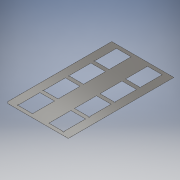
# Autodesk Inventor part: Assembly Stencil
Saved by Autodesk Inventor 2019.4 (Build 234330000, 330)
## iProperties
Created: 2021-01-11
Part Number: Assembly Stencil
Material: Stainless Steel
Document SubType Name: Modeling
Designer: caleb
Density: 8 g/cm^3
Appearance: Semi-Polished
Author: caleb
Autodesk Inventor part; units mm, degrees
ref_plane "YZ Plane" through (0, 0, 0) normal (1, 0, 0) x (0, 1, 0)
ref_plane "XZ Plane" through (0, 0, 0) normal (0, 1, 0) x (-1, 0, 0)
ref_plane "XY Plane" through (0, 0, 0) normal (0, 0, 1) x (1, 0, 0)
sketch "Sketch1" plane through (0, 0, 0) normal (0, 1, 0) x (-1, 0, 0)
  line L0 (-63.5, 107.95) -> (63.5, 107.95)
  line L1 (63.5, 107.95) -> (63.5, -107.95)
  line L2 (63.5, -107.95) -> (-63.5, -107.95)
  line L3 (-63.5, -107.95) -> (-63.5, 107.95)
  line L4 (-63.5, 107.95) -> (63.5, -107.95) construction
  line L5 (63.5, 107.95) -> (-63.5, -107.95) construction
  point P0 (0, 0)
  dimension "d0" = 215.9
  dimension "d1" = 127
  constraints: 12 end point, 2 midpoint, 2 parallel, 1 horizontal, 1 perpendicular
  measures "d0" distance of L0.end L1.end
  measures "d1" distance of L0.start L0.end
extrude "Extrusion1" add sketch "Sketch1" along normal blind 0.1
sketch "Sketch2" plane through (0, 0.1, 0) normal (0, 1, 0) x (1, 0, 0)
  line L0 (-46.5614, -100.75) -> (-16.9614, -100.75)
  line L1 (-16.7614, -100.55) -> (-16.7614, -55.95)
  line L2 (-16.9614, -55.75) -> (-46.5614, -55.75)
  line L3 (-46.7614, -55.95) -> (-46.7614, -100.55)
  line L4 (-63.5, -107.95) -> (63.5, -107.95) projected
  line L5 (-63.5, 107.95) -> (-63.5, -107.95) projected
  circle A0 centre (-46.7614, -100.75) radius 1
  arc A1 (-46.5614, -55.75) -> (-46.7614, -55.95) centre (-46.5614, -55.95) ccw
  arc A2 (-16.7614, -55.95) -> (-16.9614, -55.75) centre (-16.9614, -55.95) ccw
  arc A3 (-16.9614, -100.75) -> (-16.7614, -100.55) centre (-16.9614, -100.55) ccw
  arc A4 (-46.7614, -100.55) -> (-46.5614, -100.75) centre (-46.5614, -100.55) ccw
  arc A5 (-16.9614, -48.55) -> (-16.7614, -48.35) centre (-16.9614, -48.35) ccw
  line L6 (-16.7614, -48.35) -> (-16.7614, -3.75)
  arc A6 (-16.7614, -3.75) -> (-16.9614, -3.55) centre (-16.9614, -3.75) ccw
  line L7 (-46.5614, -48.55) -> (-16.9614, -48.55)
  arc A7 (-46.7614, -48.35) -> (-46.5614, -48.55) centre (-46.5614, -48.35) ccw
  line L8 (-16.9614, -3.55) -> (-46.5614, -3.55)
  arc A8 (-46.5614, -3.55) -> (-46.7614, -3.75) centre (-46.5614, -3.75) ccw
  line L9 (-46.7614, -3.75) -> (-46.7614, -48.35)
  arc A9 (-16.9614, 3.65) -> (-16.7614, 3.85) centre (-16.9614, 3.85) ccw
  line L10 (-16.7614, 3.85) -> (-16.7614, 48.45)
  arc A10 (-16.7614, 48.45) -> (-16.9614, 48.65) centre (-16.9614, 48.45) ccw
  line L11 (-46.5614, 3.65) -> (-16.9614, 3.65)
  arc A11 (-46.7614, 3.85) -> (-46.5614, 3.65) centre (-46.5614, 3.85) ccw
  line L12 (-16.9614, 48.65) -> (-46.5614, 48.65)
  arc A12 (-46.5614, 48.65) -> (-46.7614, 48.45) centre (-46.5614, 48.45) ccw
  line L13 (-46.7614, 48.45) -> (-46.7614, 3.85)
  arc A13 (-16.9614, 55.85) -> (-16.7614, 56.05) centre (-16.9614, 56.05) ccw
  line L14 (-16.7614, 56.05) -> (-16.7614, 100.65)
  arc A14 (-16.7614, 100.65) -> (-16.9614, 100.85) centre (-16.9614, 100.65) ccw
  line L15 (-46.5614, 55.85) -> (-16.9614, 55.85)
  arc A15 (-46.7614, 56.05) -> (-46.5614, 55.85) centre (-46.5614, 56.05) ccw
  line L16 (-16.9614, 100.85) -> (-46.5614, 100.85)
  arc A16 (-46.5614, 100.85) -> (-46.7614, 100.65) centre (-46.5614, 100.65) ccw
  line L17 (-46.7614, 100.65) -> (-46.7614, 56.05)
  arc A17 (46.5386, -100.75) -> (46.7386, -100.55) centre (46.5386, -100.55) ccw
  line L18 (46.7386, -100.55) -> (46.7386, -55.95)
  arc A18 (46.7386, -55.95) -> (46.5386, -55.75) centre (46.5386, -55.95) ccw
  line L19 (16.9386, -100.75) -> (46.5386, -100.75)
  arc A19 (16.7386, -100.55) -> (16.9386, -100.75) centre (16.9386, -100.55) ccw
  line L20 (46.5386, -55.75) -> (16.9386, -55.75)
  arc A20 (16.9386, -55.75) -> (16.7386, -55.95) centre (16.9386, -55.95) ccw
  line L21 (16.7386, -55.95) -> (16.7386, -100.55)
  arc A21 (46.5386, -48.55) -> (46.7386, -48.35) centre (46.5386, -48.35) ccw
  line L22 (46.7386, -48.35) -> (46.7386, -3.75)
  arc A22 (46.7386, -3.75) -> (46.5386, -3.55) centre (46.5386, -3.75) ccw
  line L23 (16.9386, -48.55) -> (46.5386, -48.55)
  arc A23 (16.7386, -48.35) -> (16.9386, -48.55) centre (16.9386, -48.35) ccw
  line L24 (46.5386, -3.55) -> (16.9386, -3.55)
  arc A24 (16.9386, -3.55) -> (16.7386, -3.75) centre (16.9386, -3.75) ccw
  line L25 (16.7386, -3.75) -> (16.7386, -48.35)
  arc A25 (46.5386, 3.65) -> (46.7386, 3.85) centre (46.5386, 3.85) ccw
  line L26 (46.7386, 3.85) -> (46.7386, 48.45)
  arc A26 (46.7386, 48.45) -> (46.5386, 48.65) centre (46.5386, 48.45) ccw
  line L27 (16.9386, 3.65) -> (46.5386, 3.65)
  arc A27 (16.7386, 3.85) -> (16.9386, 3.65) centre (16.9386, 3.85) ccw
  line L28 (46.5386, 48.65) -> (16.9386, 48.65)
  arc A28 (16.9386, 48.65) -> (16.7386, 48.45) centre (16.9386, 48.45) ccw
  line L29 (16.7386, 48.45) -> (16.7386, 3.85)
  arc A29 (46.5386, 55.85) -> (46.7386, 56.05) centre (46.5386, 56.05) ccw
  line L30 (46.7386, 56.05) -> (46.7386, 100.65)
  arc A30 (46.7386, 100.65) -> (46.5386, 100.85) centre (46.5386, 100.65) ccw
  line L31 (16.9386, 55.85) -> (46.5386, 55.85)
  arc A31 (16.7386, 56.05) -> (16.9386, 55.85) centre (16.9386, 56.05) ccw
  line L32 (46.5386, 100.85) -> (16.9386, 100.85)
  arc A32 (16.9386, 100.85) -> (16.7386, 100.65) centre (16.9386, 100.65) ccw
  line L33 (16.7386, 100.65) -> (16.7386, 56.05)
  circle A33 centre (-46.7614, -48.55) radius 1
  circle A34 centre (-46.7614, 3.65) radius 1
  circle A35 centre (-46.7614, 55.85) radius 1
  circle A36 centre (46.736, -100.75) radius 1
  circle A37 centre (46.736, -48.55) radius 1
  circle A38 centre (46.736, 3.65) radius 1
  circle A39 centre (46.736, 55.85) radius 1
  line L34 (63.5, -107.95) -> (63.5, 107.95) projected
  point P0 (0, 0)
  point P1 (-16.7614, -100.75)
  point P2 (-46.7614, -55.75)
  point P3 (-16.7614, -48.55)
  point P4 (-46.7614, -3.55)
  point P5 (-16.7614, 3.65)
  point P6 (-46.7614, 48.65)
  point P7 (-16.7614, 55.85)
  point P8 (-46.7614, 100.85)
  point P9 (46.7386, -100.75)
  point P10 (16.7386, -100.75)
  point P11 (16.7386, -100.75)
  point P12 (16.7386, -55.75)
  point P13 (46.7386, -48.55)
  point P14 (16.7386, -48.55)
  point P15 (16.7386, -48.55)
  point P16 (16.7386, -3.55)
  point P17 (46.7386, 3.65)
  point P18 (16.7386, 3.65)
  point P19 (16.7386, 3.65)
  point P20 (16.7386, 48.65)
  point P21 (46.7386, 55.85)
  point P22 (16.7386, 55.85)
  point P23 (16.7386, 55.85)
  point P24 (16.7386, 100.85)
  dimension "d4" = 30
  dimension "d5" = 45
  dimension "d6" = 7.2
  dimension "d7" = 16.7386
  dimension "d8" = 2
  dimension "d9" = 0.2
  dimension "d20" = 0.2
  dimension "d23" = 52.2
  dimension "d26" = 63.5
  dimension "d31" = 52.2
  dimension "d34" = 93.4974
  dimension "d37" = 16.7614
  constraints: 64 end point, 64 point on circle, 48 point on line, 40 centre point, 8 coincident, 8 tangent, 3 horizontal, 2 equal radius, 2 parallel, 2 vertical, 1 perpendicular, 182 other
  measures "d4" distance of point (-46.761, -100.75) point (-16.761, -100.75)
  measures "d5" distance of point (-46.761, -55.75) point (-46.761, -100.75)
  measures "d6" distance between parallel lines of L4 L0
  measures "d7" distance between parallel lines of L5 L3
  measures "d8" diameter of A0
  measures "d9" radius of A1
  measures "d20" radius of A4
  measures "d23" distance of point (-16.761, -100.75) point (-16.761, -48.55)
  measures "d26" distance of point (-16.761, -100.75) point (46.739, -100.75)
  measures "d31" distance of A0.centre A33.centre
  measures "d34" distance of A0.centre A36.centre
  measures "d37" distance between parallel lines of L34 L18
extrude "Extrusion2" cut sketch "Sketch2" against normal through all
chamfer "Chamfer1" distance 3.175 angle 45 1 edges at (-63.5, 0.05, 107.95)
body "Solid1"
